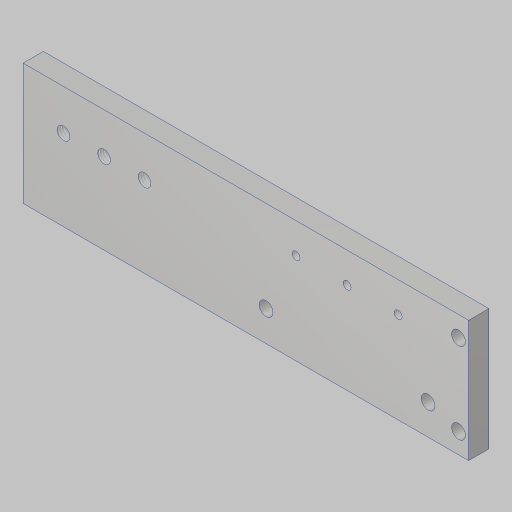
# Autodesk Inventor part: EL2-021
Saved by Autodesk Inventor 2023.5 (Build 275446000, 446)
## iProperties
Created: 2025-01-21
Part Number: EL2-021
Material: Aluminum 6061
Document SubType Name: Modeling
Designer: slick
Density: 2.7 g/cm^3
Appearance: Aluminum - Flat
Author: slick
Autodesk Inventor part; units mm, degrees
ref_plane "YZ Plane" through (0, 0, 0) normal (1, 0, 0) x (0, 1, 0)
ref_plane "XZ Plane" through (0, 0, 0) normal (0, 1, 0) x (-1, 0, 0)
ref_plane "XY Plane" through (0, 0, 0) normal (0, 0, 1) x (1, 0, 0)
sketch "Sketch1" plane through (0, 0, 0) normal (0, 0, 1) x (1, 0, 0)
  line L0 (69.85, -19.05) -> (-69.85, -19.05)
  line L1 (-69.85, -19.05) -> (-69.85, 19.05)
  line L2 (-69.85, 19.05) -> (69.85, 19.05)
  line L3 (69.85, 19.05) -> (69.85, -19.05)
  line L4 (69.85, -19.05) -> (-69.85, 19.05) construction
  line L5 (-69.85, -19.05) -> (69.85, 19.05) construction
  point P0 (0, 0)
  dimension "d0" = 139.7
  dimension "d1" = 38.1
  constraints: 12 end point, 2 midpoint, 2 parallel, 1 horizontal, 1 perpendicular
  measures "d0" distance of L1.end L2.end
  measures "d1" distance of L0.end L1.end
extrude "Extrusion1" add sketch "Sketch1" along normal blind 6.35
sketch "Sketch2" plane through (0, 0, 6.35) normal (0, 0, 1) x (1, 0, 0)
  line L0 (-69.85, 19.05) -> (-69.85, -19.05) projected
  line L1 (69.85, 19.05) -> (-69.85, 19.05) projected
  point P0 (0, 0)
  point P1 (-57.15, 6.35)
  point P2 (-44.45, 6.35)
  point P3 (-31.75, 6.35)
  point P4 (-69.85, 0)
  dimension "d5" = 12.7
  dimension "d6" = 12.7
  dimension "d14" = 12.7
  dimension "d15" = 12.7
  constraints: 2 horizontal alignment, 1 midpoint
  measures "d5" distance of point (-44.45, 6.35) point (-57.15, 6.35)
  measures "d6" distance of point (-44.45, 6.35) point (-31.75, 6.35)
  measures "d14" distance from line of L1 point (-57.15, 6.35)
  measures "d15" distance from line of L0 point (-57.15, 6.35)
hole "Hole1" at (-57.15, 6.35, 6.35) at (-44.45, 6.35, 6.35) at (-31.75, 6.35, 6.35) direction (0, 0, -1) diameter 3.9624 end through all thread size "10-32 UNF" class "2B" standard "ANSI Unified Screw Threads"
sketch "Sketch3" plane through (0, 0, 6.35) normal (0, 0, 1) x (1, 0, 0)
  line L0 (69.85, 19.05) -> (-69.85, 19.05) projected
  line L1 (-69.85, -19.05) -> (69.85, -19.05) projected
  line L2 (69.85, -19.05) -> (69.85, 19.05) projected
  line L3 (6.35, -9.525) -> (57.15, -9.525) construction
  line L4 (-69.85, 19.05) -> (-69.85, -19.05) construction
  point P0 (0, 0)
  point P1 (66.675, 12.7)
  point P2 (66.675, -12.7)
  point P3 (-69.85, 0)
  dimension "d16" = 6.35
  dimension "d17" = 6.35
  dimension "d18" = 3.175
  dimension "d39" = 50.8
  dimension "d41" = 28.575
  dimension "d43" = 12.7
  constraints: 2 end point, 1 horizontal, 1 midpoint, 1 vertical alignment
  measures "d16" distance from line of L0 point (66.675, 12.7)
  measures "d17" distance from line of L1 point (66.675, -12.7)
  measures "d18" distance from line of L2 point (66.675, 12.7)
  measures "d39" distance of L3.start L3.end
  measures "d41" distance between parallel lines of L0 L3
  measures "d43" distance from line of L2 L3.end
hole "Hole2" at (66.675, 12.7, 6.35) at (66.675, -12.7, 6.35) at (6.35, -9.525, 6.35) at (57.15, -9.525, 6.35) direction (0, 0, -1) diameter 4.318 end through all clearance for "Flat Head Machine Screw (82)" size "#8" standard "Ansi Unified Screw Threads"
sketch "Sketch6" plane through (0, 0, 6.35) normal (0, 0, 1) x (1, 0, 0)
  line L0 (47.75, 9.525) -> (15.75, 9.525) construction
  line L1 (69.85, -19.05) -> (69.85, 19.05) construction
  line L2 (-69.85, -19.05) -> (69.85, -19.05) construction
  point P0 (0, 0)
  point P1 (69.85, 0)
  point P2 (69.85, 0)
  point P3 (31.75, 9.525)
  point P4 (31.75, 1.524)
  dimension "d30" = 32
  dimension "d45" = 28.575
  dimension "d46" = 38.1
  dimension "d47" = 8.001
  constraints: 3 midpoint, 2 end point, 1 horizontal, 1 vertical alignment
  measures "d30" distance of L0.start L0.end
  measures "d45" distance between parallel lines of L0 L2
  measures "d46" distance from line of L1 point (31.75, 9.525)
  measures "d47" distance from line of point (31.75, 1.524) L0
hole "Hole3" at (47.75, 9.525, 6.35) at (15.75, 9.525, 6.35) at (31.75, 9.525, 6.35) direction (0, 0, -1) diameter 2.459 end through all thread size "M3x0.5" class "6H" standard "ANSI Metric M Profile"
equation "\"d5\" = d4"
equation "\"d6\" = d4"
equation "\"d4\" = 12.7"
body "Solid1"
